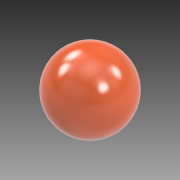
# Autodesk Inventor part: FRC 2010 Ball
Saved by Autodesk Inventor 2022 (Build 260153000, 153)
## iProperties
Created: 2021-05-01
Part Number: FRC 2010 Ball
Material: Generic
Document SubType Name: Modeling
Designer: Cal
Mass: 396.893 g
Surface Area: 1551.79 cm^2
Volume: 5748.09 cm^3
Density: 0.0690478 g/cm^3
Appearance: Smooth - Light Orange
Author: Cal
Autodesk Inventor part; units mm, degrees
ref_plane "YZ Plane" through (0, 0, 0) normal (1, 0, 0) x (0, 1, 0)
ref_plane "XZ Plane" through (0, 0, 0) normal (0, 1, 0) x (-1, 0, 0)
ref_plane "XY Plane" through (0, 0, 0) normal (0, 0, 1) x (1, 0, 0)
sketch "Sketch1" plane through (0, 0, 0) normal (0, 0, 1) x (1, 0, 0)
  arc A0 (0, -101.6) -> (0, 101.6) centre (0, 0) ccw
  line L0 (0, 101.6) -> (0, -101.6)
  dimension "d0" = 203.2
  constraints: 2 end point, 2 point on circle, 1 centre point, 1 coincident, 1 midpoint, 1 vertical
  measures "d0" diameter of A0
revolve "Revolution1" add sketch "Sketch1" angle 360 about axis through (0, 101.6, 0) along (0, -1, 0)
body "Solid1"
